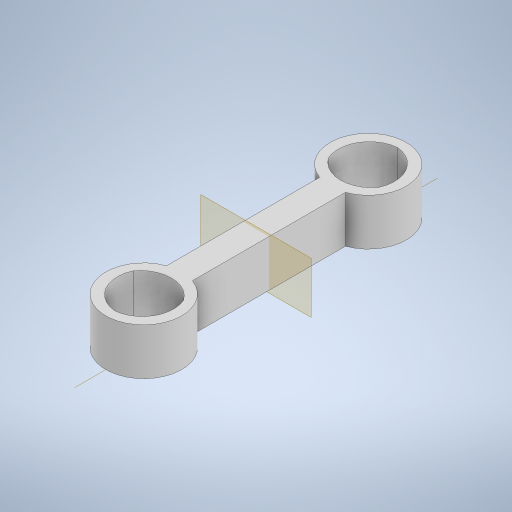
# Autodesk Inventor part: Knochen13
Saved by Autodesk Inventor 2023 (Build 270158000, 158)
## iProperties
Created: 2023-07-06
Part Number: Knochen13
Material: Generisch
Document SubType Name: Modeling
Designer: prigge
Density: 1 g/cm^3
Appearance: Vorgabe
Author: prigge
Autodesk Inventor part; units mm, degrees
ref_plane "YZ Plane" through (0, 0, 0) normal (1, 0, 0) x (0, 1, 0)
ref_plane "XZ Plane" through (0, 0, 0) normal (0, 1, 0) x (-1, 0, 0)
sketch "Skizze1" plane through (0, 0, 0) normal (0, 1, 0) x (-1, 0, 0)
  circle A0 centre (0, 0) radius 1.7
  circle A1 centre (0, -13) radius 1.7
  line L0 (0, -18.68) -> (0, 5.68) projected
  circle A2 centre (0, -13) radius 2.2
  circle A3 centre (0, 0) radius 2.2
  line L1 (-0.75, -10.9318) -> (-0.75, -2.0682)
  line L2 (0.75, -10.9318) -> (0.75, -2.0682)
  dimension "d0" = 3.4
  dimension "d2" = 13
  dimension "d3" = 1.5
  dimension "d4" = 4.4
  constraints: 4 centre point, 4 end point, 4 point on circle, 3 coincident, 2 equal radius, 1 parallel, 1 point on line, 1 vertical, 1 other
  measures "d0" diameter of A1
  measures "d2" distance of point (0, 0) A1.centre
  measures "d3" distance between parallel lines of L1 L2
  measures "d4" diameter of A2
extrude "Extrusion1" add sketch "Skizze1" along normal blind 2.7 contours A0 L0 A3 | A0 L0 A3 | A3 L2 A2 L0 | L0 A2 L1 A3 | A2 L0 A1 | L0 A1 A2
sketch "Skizze3" plane through (0, 0, 0) normal (0, 1, 0) x (-1, 0, 0)
  circle A0 centre (0, 0) radius 1.7 projected
  circle A1 centre (0, 0) radius 1.6 construction
  arc A2 (-1.5131, -0.775) -> (1.5131, -0.775) centre (0, 0.2) ccw
  arc A3 (1.4277, -0.9229) -> (-0.0854, 1.6979) centre (-0.1732, -0.1) ccw
  arc A4 (0.0854, 1.6979) -> (-1.4277, -0.9229) centre (0.1732, -0.1) ccw
  point P0 (0, -1.6)
  point P1 (1.3856, 0.8)
  point P2 (-1.3856, 0.8)
  point P3 (-0.0854, 1.6979)
  point P4 (1.4277, -0.9229)
  point P5 (-1.4277, -0.9229)
  point P6 (0.0854, 1.6979)
  dimension "d8" = 3.2
  dimension "d9" = 0.2
  dimension "d12" = 360
  constraints: 9 point on circle, 3 centre point, 1 coincident, 1 horizontal alignment, 1 vertical alignment, 18 other
  measures "d9" distance of point (0, 0) A2.centre
extrude "Extrusion2" add sketch "Skizze3" along normal up to surface (2.7 mm away) contours A0 A2 A3 A4 | A4 A3 A0 | A0 A3 A2 | A3 A4 A2 A0 | A0 A4 A2 A3 | A2 A4 A0
ref_plane "Arbeitsebene1" through (0, 0, -6.5) normal (0, 0, 1) x (1, 0, 0)
mirror "Spiegeln1" about plane through (0, 0, -6.5) normal (0, 0, 1) of "Extrusion2"
